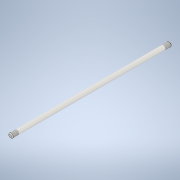
# Autodesk Inventor part: Gewindestange_360
Saved by Autodesk Inventor 2020.3 (Build 243373000, 373)
## iProperties
Created: 2021-05-20
Part Number: Gewindestange_360
Material: Stahl AISI 4130
Document SubType Name: Modeling
Designer: Preuß P. Ch.
Density: 7.85 g/cm^3
Appearance: Stahl
Author: Preuß P. Ch.
Autodesk Inventor part; units mm, degrees
ref_plane "YZ Plane" through (0, 0, 0) normal (1, 0, 0) x (0, 1, 0)
ref_plane "XZ Plane" through (0, 0, 0) normal (0, 1, 0) x (-1, 0, 0)
ref_plane "XY Plane" through (0, 0, 0) normal (0, 0, 1) x (1, 0, 0)
sketch "Skizze1" plane through (0, 0, 0) normal (0, 1, 0) x (-1, 0, 0)
  line L0 (0, 0) -> (5, 0)
  line L1 (5, 0) -> (5, -180)
  line L2 (5, -180) -> (0, -180)
  line L3 (0, -180) -> (0, 0)
  dimension "d0" = 180
  dimension "d1" = 10
  constraints: 8 end point, 2 parallel, 1 horizontal, 1 perpendicular
  measures "d0" distance of L2.end L0.start
  measures "d1" diameter of L1 L3
revolve "Umdrehung1" add sketch "Skizze1" angle 360 about axis through (0, 0, -180) along (0, 0, 1)
thread "Gewinde1" size "M10x1.5" class "6g" standard "ISO Metric profile" length 15
chamfer "Fase1" distance 2 angle 45 1 edges at (5, 0, 0)
mirror "Spiegeln1" about plane through (0, 0, -180) normal (0, 0, -1)
